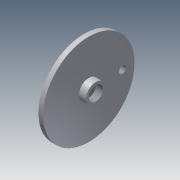
# Autodesk Inventor part: servo_paka1
Saved by Autodesk Inventor 2013 (Build 170138000, 138)
## iProperties
Created: 2013-01-27
Part Number: servo_paka1
Material: Generic
Document SubType Name: Modeling
Designer: idle-rug
Density: 1 g/cm^3
Author: idle-rug
Autodesk Inventor part; units mm, degrees
ref_plane "YZ Plane" through (0, 0, 0) normal (1, 0, 0) x (0, 1, 0)
ref_plane "XZ Plane" through (0, 0, 0) normal (0, 1, 0) x (-1, 0, 0)
ref_plane "XY Plane" through (0, 0, 0) normal (0, 0, 1) x (1, 0, 0)
sketch "Sketch1" plane through (0, 0, 0) normal (1, 0, 0) x (0, 1, 0)
  circle A0 centre (0, 0) radius 19.3
  dimension "d0" = 38.6
  constraints: 1 centre point, 1 coincident
  measures "d0" diameter of A0
extrude "Extrusion1" add sketch "Sketch1" along normal blind 2
sketch "Sketch2" plane through (2, 0, 0) normal (1, 0, 0) x (0, 0, -1)
  circle A0 centre (0, 0) radius 4.2
  dimension "d4" = 8.4
  constraints: 1 centre point
  measures "d4" diameter of A0
extrude "Extrusion2" add sketch "Sketch2" along normal blind 3
sketch "Sketch4" plane through (5, 0, 0) normal (1, 0, 0) x (0, 0, -1)
  circle A0 centre (0, 0) radius 4.2 projected
  circle A1 centre (0, 0) radius 3
  dimension "d7" = 6
  constraints: 1 centre point, 1 coincident
  measures "d7" diameter of A1
extrude "Extrusion3" cut sketch "Sketch4" against normal blind 3 contours A1
sketch "Sketch5" plane through (0, 0, 0) normal (-1, 0, 0) x (0, 0, 1)
  circle A0 centre (0, 14.25) radius 1.5
  dimension "d11" = 3
  constraints: 1 centre point
  measures "d11" diameter of A0
extrude "Extrusion4" cut sketch "Sketch5" against normal blind 2
body "Solid1"
